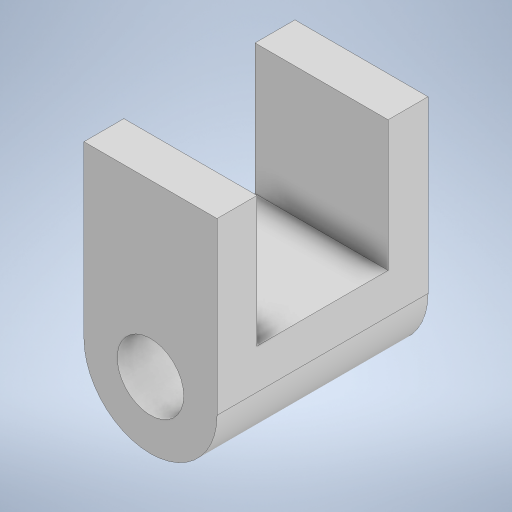
# Autodesk Inventor part: Part2
Saved by Autodesk Inventor 2024 (Build 280153000, 153)
## iProperties
Created: 2023-06-11
Part Number: Part2
Material: Generic
Document SubType Name: Modeling
Designer: dipes
Density: 1 g/cm^3
Appearance: Default
Author: dipes
Autodesk Inventor part; units mm, degrees
ref_plane "YZ Plane" through (0, 0, 0) normal (1, 0, 0) x (0, 1, 0)
ref_plane "XZ Plane" through (0, 0, 0) normal (0, 1, 0) x (-1, 0, 0)
ref_plane "XY Plane" through (0, 0, 0) normal (0, 0, 1) x (1, 0, 0)
sketch "Sketch2" plane through (0, 0, 0) normal (0, 0, 1) x (1, 0, 0)
  line L0 (0, 0) -> (0, 6)
  line L1 (20, 6) -> (20, 0)
  line L2 (20, 0) -> (0, 0)
  line L3 (10, 0) -> (10, 9.1281) construction
  arc A0 (0, 0) -> (20, 0) centre (10, 0) ccw
  circle A1 centre (10, 0) radius 5
  line L4 (0, 6) -> (20, 6)
  point P0 (20, 0)
  dimension "d14" = 20
  dimension "d15" = 10
  dimension "d18" = 6
  dimension "d19" = 20
  dimension "d20" = 6
  constraints: 10 end point, 2 centre point, 2 coincident, 2 perpendicular, 2 point on circle, 2 point on line, 2 vertical, 1 midpoint
  measures "d14" diameter of A0
  measures "d15" diameter of A1
  measures "d18" distance of L0.start L0.end
  measures "d19" distance of L0.end L1.start
  measures "d20" distance of L1.start L1.end
extrude "Extrusion2" add sketch "Sketch2" along normal blind 31.7 contours L0 L4 L1 L2 A1 | L2 A1 A0
sketch "Sketch3" plane through (0, 6, 0) normal (0, 1, 0) x (1, 0, 0)
  line L0 (20, 0) -> (20, -31.7) projected
  line L1 (0, 0) -> (20, 0)
  line L2 (20, 0) -> (20, -6)
  line L3 (20, -6) -> (0, -6)
  line L4 (0, -6) -> (0, 0)
  line L5 (20, -31.7) -> (0, -31.7) projected
  line L6 (0, -31.7) -> (20, -31.7)
  line L7 (20, -31.7) -> (20, -25.7)
  line L8 (20, -25.7) -> (0, -25.7)
  line L9 (0, -25.7) -> (0, -31.7)
  dimension "d21" = 6
  dimension "d22" = 6
  constraints: 16 end point, 4 parallel, 2 horizontal, 2 perpendicular, 2 point on line
  measures "d21" distance of L1.end L2.end
  measures "d22" distance of L7.end L6.end
extrude "Extrusion3" add sketch "Sketch3" along normal blind 19.6
body "Solid2"
